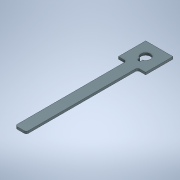
# Autodesk Inventor part: pb_hole_stick
Saved by Autodesk Inventor 2021 (Build 250183000, 183)
## iProperties
Created: 2022-02-27
Part Number: pb_hole_stick
Material: Lead
Document SubType Name: Modeling
Designer: ermoz
Density: 11.34 g/cm^3
Appearance: Lead
Mass: 12.3267 g
Surface Area: 13.3642 cm^2
Volume: 1.08701 cm^3
Author: ermoz
Autodesk Inventor part; units mm, degrees
ref_plane "YZ Plane" through (0, 0, 0) normal (1, 0, 0) x (0, 1, 0)
ref_plane "XZ Plane" through (0, 0, 0) normal (0, 1, 0) x (-1, 0, 0)
ref_plane "XY Plane" through (0, 0, 0) normal (0, 0, 1) x (1, 0, 0)
sketch "Sketch1" plane through (0, 0, 0) normal (0, 1, 0) x (-1, 0, 0)
  circle A0 centre (0, 0) radius 4.25
  line L0 (-12.25, -12.25) -> (12.25, -12.25)
  line L1 (12.25, -12.25) -> (12.25, 12.25)
  line L2 (12.25, 12.25) -> (-12.25, 12.25)
  line L3 (-12.25, 12.25) -> (-12.25, -12.25)
  line L4 (-12.25, -12.25) -> (12.25, 12.25) construction
  line L5 (12.25, -12.25) -> (-12.25, 12.25) construction
  dimension "d0" = 24.5
  dimension "d1" = 8.5
  constraints: 12 end point, 2 midpoint, 2 parallel, 2 perpendicular, 1 centre point, 1 coincident, 1 horizontal
  measures "d0" distance of L0.start L0.end
  measures "d1" diameter of A0
extrude "Extrusion1" add sketch "Sketch1" along normal blind 2
sketch "Sketch2" plane through (0, 2, 0) normal (0, 1, 0) x (1, 0, 0)
  circle A0 centre (0, -4.9582) radius 1.5
  point P0 (0, 0)
  dimension "d4" = 3
  constraints: 1 centre point
  measures "d4" diameter of A0
extrude "Extrusion2" cut sketch "Sketch2" against normal blind 3
sketch "Sketch3" plane through (0, 2, 0) normal (0, 1, 0) x (1, 0, 0)
  line L0 (-12.25, -12.25) -> (12.25, -12.25) projected
  line L1 (5, -112.25) -> (-5, -112.25)
  line L2 (-5, -112.25) -> (-5, -12.25)
  line L3 (-5, -12.25) -> (5, -12.25)
  line L4 (5, -12.25) -> (5, -112.25)
  line L5 (5, -112.25) -> (-5, -12.25) construction
  line L6 (-5, -112.25) -> (5, -12.25) construction
  point P0 (0, 0)
  point P1 (0, -62.25)
  point P2 (0, -62.25)
  point P3 (5, -12.25)
  dimension "d7" = 100
  dimension "d8" = 10
  constraints: 12 end point, 3 midpoint, 2 parallel, 1 horizontal, 1 perpendicular, 1 point on line, 1 vertical alignment
  measures "d7" distance of L3.end L1.start
  measures "d8" distance between parallel lines of L2 L4
extrude "Extrusion3" add sketch "Sketch3" against normal up to surface (2 mm away)
fillet "Fillet1" radius 2 4 edges at (5, 1, 12.25) (-5, 1, 12.25) (5, 1, 112.25) (-5, 1, 112.25)
equation "\"d5\" = d4"
body "Solid1"
